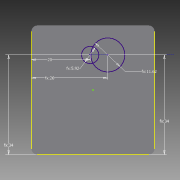
# Autodesk Inventor part: wall-middle
Saved by Autodesk Inventor 2015 (Build 190159000, 159)
## iProperties
Created: 2014-07-16
Part Number: wall-middle
Material: Generic
Document SubType Name: Modeling
Designer: pc
Density: 1 g/cm^3
Appearance: Default
Author: pc
Autodesk Inventor part; units mm, degrees
ref_plane "YZ Plane" through (0, 0, 0) normal (1, 0, 0) x (0, 1, 0)
ref_plane "XZ Plane" through (0, 0, 0) normal (0, 1, 0) x (-1, 0, 0)
ref_plane "XY Plane" through (0, 0, 0) normal (0, 0, 1) x (1, 0, 0)
sketch "Sketch1" plane through (0, 0, 0) normal (0, 1, 0) x (-1, 0, 0)
  line L0 (-21, 22) -> (21, 22)
  line L1 (21, 22) -> (21, -22)
  line L2 (21, -22) -> (-21, -22)
  line L3 (-21, -22) -> (-21, 22)
  line L4 (-21, 22) -> (21, -22) construction
  line L5 (21, 22) -> (-21, -22) construction
  point P0 (0, 0)
  dimension "d0" = 42
  dimension "d1" = 44
  constraints: 12 end point, 2 midpoint, 2 parallel, 1 horizontal, 1 perpendicular
  measures "d0" distance of L1.end L2.end
  measures "d1" distance of L0.end L1.end
extrude "Extrusion1" add sketch "Sketch1" along normal blind 6.4
fillet "Fillet1" radius 2 2 edges at (-21, 3.2, 22) (21, 3.2, 22)
fillet "Fillet2" radius 2 1 edges at (21, 3.2, -22)
fillet "Fillet3" radius 2 1 edges at (-21, 3.2, -22)
sketch "Servobigcircle" plane through (0, 6.4, 0) normal (0, 1, 0) x (1, 0, 0)
  circle A0 centre (5, 12) radius 5.81
  line L0 (21, -20) -> (21, 20) projected
  line L1 (-21, 20) -> (-21, -20) projected
  line L2 (-19, -22) -> (19, -22) projected
  line L3 (27.852, 12) -> (-23.8048, 12) construction
  dimension "d7" = 11.62
  dimension "d12" = 26
  dimension "d13" = 34
  constraints: 2 end point, 1 centre point, 1 horizontal, 1 point on line
  measures "d7" diameter of A0
  measures "d12" distance from line of L1 A0.centre
  measures "d13" distance from line of L2 A0.centre
sketch "servosmall" plane through (0, 6.4, 0) normal (0, 1, 0) x (1, 0, 0)
  line L0 (-21, 20) -> (-21, -20) projected
  circle A0 centre (-1, 12) radius 2.96
  line L1 (-19, -22) -> (19, -22) projected
  point P0 (0, 0)
  dimension "d26" = 20
  dimension "d28" = 34
  dimension "d29" = 5.92
  constraints: 1 centre point
  measures "d26" distance from line of L0 A0.centre
  measures "d28" distance from line of L1 A0.centre
  measures "d29" diameter of A0
equation "\"d0\" = wallw"
equation "\"d1\" = wallh"
equation "\"d2\" = wall2_thick"
equation "\"d4\" = cornerrad"
equation "\"d5\" = cornerrad"
equation "\"d6\" = cornerrad"
equation "\"d7\" = servobigcircledia"
equation "\"d12\" = distancefromleft"
equation "\"d13\" = distancefrombottom"
equation "\"d28\" = d13"
equation "\"d29\" = servosmallcircledia"
equation "\"printer3dtolerance\" = 0.12"
equation "\"wallw\" = 42"
equation "\"wallh\" = 44"
equation "\"cornerrad\" = 2"
equation "\"baseextra\" = 2"
equation "\"wall1_thick\" = 8"
equation "\"wall2_thick\" = 6.4"
equation "\"wall3_thick\" = 4"
equation "\"wall1slot\" = 8.12"
equation "\"wall2slot\" = 6.52"
equation "\"wall3slot\" = 4.12"
equation "\"gap2\" = 28"
equation "\"baseh\" = 79.12"
equation "\"basew\" = 44"
equation "\"base_thick\" = 6"
equation "\"base_slots_depth\" = 4"
equation "\"servomounth\" = 4"
equation "\"servosmallcircledia\" = 5.92"
equation "\"servomountsquare\" = 6"
equation "\"servobigcircledia\" = 11.62"
equation "\"servo9gw\" = 22.8"
equation "\"distancefromleft\" = 26"
equation "\"servopolygonl\" = 5.92"
equation "\"servopolygonr\" = 6.12"
equation "\"distancefrombottom\" = 34"
body "Solid1"
